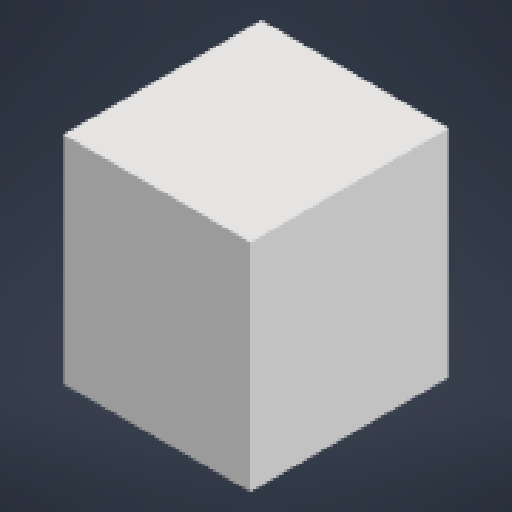
# Autodesk Inventor part: Down Right Building Block
Saved by Autodesk Inventor 2024 (Build 280153000, 153)
## iProperties
Created: 2023-06-19
Part Number: Down Right Building Block
Material: Glass
Document SubType Name: Modeling
Designer: juanj
Density: 2.18 g/cm^3
Appearance: Clear
Author: juanj
Autodesk Inventor part; units mm, degrees
ref_plane "YZ Plane" through (0, 0, 0) normal (1, 0, 0) x (0, 1, 0)
ref_plane "XZ Plane" through (0, 0, 0) normal (0, 1, 0) x (-1, 0, 0)
ref_plane "XY Plane" through (0, 0, 0) normal (0, 0, 1) x (1, 0, 0)
sketch "Sketch1" plane through (0, 0, 0) normal (0, 0, 1) x (1, 0, 0)
  line L0 (0, 0) -> (104, 0)
  line L1 (104, 0) -> (104, 120)
  line L2 (104, 120) -> (0, 120)
  line L3 (0, 120) -> (0, 0)
  dimension "d0" = 104
  dimension "d1" = 120
  constraints: 8 end point, 2 parallel, 1 horizontal, 1 perpendicular
  measures "d0" distance of L2.end L1.end
  measures "d1" distance of L1.end L0.end
extrude "Extrusion1" add sketch "Sketch1" along normal blind 110
body "Solid1"
